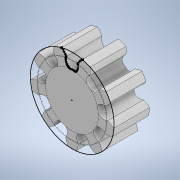
# Autodesk Inventor part: SmallGear9T
Saved by Autodesk Inventor 2022 (Build 260153070, 153G)
## iProperties
Created: 2021-11-03
Part Number: SmallGear9T
Material: Generic
Document SubType Name: Modeling
Designer: a laptop
Density: 1 g/cm^3
Appearance: Default
Author: a laptop
Autodesk Inventor part; units mm, degrees
ref_plane "YZ Plane" through (0, 0, 0) normal (1, 0, 0) x (0, 1, 0)
ref_plane "XZ Plane" through (0, 0, 0) normal (0, 1, 0) x (-1, 0, 0)
ref_plane "XY Plane" through (0, 0, 0) normal (0, 0, 1) x (1, 0, 0)
sketch "Sketch1" plane through (0, 0, 0) normal (0, 0, 1) x (1, 0, 0)
  spline S0 degree 3 poles (-0.8759, 3.3893) (-0.8383, 3.3556) (-0.7633, 3.2881) (-0.6628, 3.1749) (-0.5715, 3.0536) (-0.5266, 2.9632) (-0.5041, 2.918) knots 0 0 0 0 0.015124 0.030247 0.045369 0.06048 0.06048 0.06048 0.06048
  spline S1 degree 3 poles (-0.5041, 2.918) (-0.5109, 2.8742) (-0.5246, 2.7867) (-0.5232, 2.6535) (-0.5053, 2.5216) (-0.4672, 2.4165) (-0.4203, 2.3413) (-0.3774, 2.2903) (-0.3247, 2.2492) (-0.2647, 2.22) (-0.1992, 2.2046) (-0.1104, 2.2098) (0, 2.2141) (0.1104, 2.2098) (0.1992, 2.2046) (0.2647, 2.22) (0.3247, 2.2492) (0.3774, 2.2903) (0.4203, 2.3413) (0.4672, 2.4165) (0.5053, 2.5216) (0.5232, 2.6535) (0.5246, 2.7867) (0.5109, 2.8742) (0.5041, 2.918) knots 0 0 0 0 0.013267 0.026535 0.039801 0.053056 0.059681 0.066311 0.072942 0.079573 0.086209 0.092853 0.106117 0.119382 0.126026 0.132662 0.139292 0.145924 0.152553 0.159179 0.172433 0.185699 0.198967 0.212234 0.212234 0.212234 0.212234
  spline S2 degree 3 poles (0.5041, 2.918) (0.5266, 2.9632) (0.5715, 3.0536) (0.6628, 3.1749) (0.7633, 3.2881) (0.8383, 3.3556) (0.8759, 3.3893) knots 0 0 0 0 0.015111 0.030233 0.045356 0.06048 0.06048 0.06048 0.06048
  circle A0 centre (0, 0) radius 2.2124 construction
  circle A1 centre (0, 0) radius 2.8806 construction
  circle A2 centre (0, 0) radius 2.925 construction
  circle A3 centre (0, 0) radius 3.5007
  point P0 (-0.7653, 3.2861)
  point P1 (-0.6643, 3.1735)
  point P2 (-0.5755, 3.0512)
  point P3 (-0.521, 2.7864)
  point P4 (-0.5205, 2.6537)
  point P5 (-0.5007, 2.5225)
  point P6 (-0.4541, 2.3984)
  point P7 (-0.419, 2.3422)
  point P8 (-0.3758, 2.292)
  point P9 (-0.3235, 2.2512)
  point P10 (-0.2638, 2.2223)
  point P11 (-0.199, 2.2078)
  point P12 (-0.1326, 2.2083)
  point P13 (0, 2.2124)
  point P14 (0.1326, 2.2083)
  point P15 (0.199, 2.2078)
  point P16 (0.2638, 2.2223)
  point P17 (0.3235, 2.2512)
  point P18 (0.3758, 2.292)
  point P19 (0.419, 2.3422)
  point P20 (0.4541, 2.3984)
  point P21 (0.5007, 2.5225)
  point P22 (0.5205, 2.6537)
  point P23 (0.521, 2.7864)
  point P24 (0.5755, 3.0512)
  point P25 (0.6643, 3.1735)
  point P26 (0.7653, 3.2861)
  constraints: 4 centre point, 2 point on circle, 69 other
extrude "Extrusion1" add sketch "Sketch1" against normal blind 3
extrude "Extrusion2" cut sketch "Sketch1" against normal blind 10 contours A3 S2 S1 S0 picked at (0.0983, 3.1081)
pattern_circular "Circular Pattern1" count 9 over 360 about axis through (0, 0, 0) along (0, 0, -1) of "Extrusion2"
equation "\"d0\" = FaceWidth"
equation "\"Module\" = 0.65"
equation "\"PressureAngle\" = 10deg"
equation "\"UnitProfileClearance\" = 0.25"
equation "\"UnitRoundRadius\" = 0.3025"
equation "\"HeadDiameter\" = 7.00133"
equation "\"RootDiameter\" = 4.42478"
equation "\"BaseDiameter\" = 5.76113"
equation "\"PitchDiameter\" = 5.85"
equation "\"FaceWidth\" = 3"
equation "\"HelixAngle\" = 0"
equation "\"UnitCorrection\" = 0.153676"
equation "\"UnitAddendumModification\" = 0.268038"
equation "\"CircularPitch\" = 2.04204"
equation "\"UnitBacklashShift\" = 0"
equation "\"TotalToolShift\" = 0.09989"
equation "\"IsInternal\" = 0"
body "Solid1"
